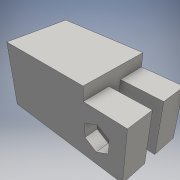
# Autodesk Inventor part: connectiontest1
Saved by Autodesk Inventor 2016 (Build 200138000, 138)
## iProperties
Created: 2015-11-19
Part Number: connectiontest1
Material: Generic
Document SubType Name: Modeling
Designer: hesaon
Density: 1 g/cm^3
Appearance: Default
Author: hesaon
Autodesk Inventor part; units mm, degrees
ref_plane "YZ Plane" through (0, 0, 0) normal (1, 0, 0) x (0, 1, 0)
ref_plane "XZ Plane" through (0, 0, 0) normal (0, 1, 0) x (-1, 0, 0)
ref_plane "XY Plane" through (0, 0, 0) normal (0, 0, 1) x (1, 0, 0)
sketch "Sketch1" plane through (0, 0, 0) normal (0, 0, 1) x (1, 0, 0)
  line L0 (0, 0) -> (-40, 0)
  line L1 (-40, 0) -> (-40, 20)
  line L2 (-40, 20) -> (0, 20)
  line L3 (0, 20) -> (0, 0)
  dimension "d0" = 40
  dimension "d1" = 20
  constraints: 8 end point, 2 parallel, 1 horizontal, 1 perpendicular
  measures "d0" distance of L1.end L2.end
  measures "d1" distance of L0.end L1.end
extrude "Extrusion1" add sketch "Sketch1" along normal blind 20
sketch "Sketch2" plane through (-40, 20, 0) normal (0, 1, 0) x (1, 0, 0)
  line L0 (0, -20) -> (40, -20) projected
  line L1 (40, -20) -> (40, -16)
  line L2 (40, 0) -> (40, -20) projected
  line L3 (28, -20) -> (28, -16)
  line L4 (28, -16) -> (40, -16)
  dimension "d4" = 4
  dimension "d5" = 12
  constraints: 6 end point, 2 point on line, 1 perpendicular, 1 vertical
  measures "d4" distance of L0.end L1.end
  measures "d5" distance of L1.end L3.end
extrude "Extrusion2" cut sketch "Sketch2" against normal through all
sketch "Sketch3" plane through (0, 0, 0) normal (1, 0, 0) x (0, 0, -1)
  line L0 (-16, 20) -> (-16, 0) projected
  line L1 (-16, 12) -> (0, 12)
  line L2 (0, 20) -> (0, 0) projected
  line L3 (0, 8) -> (-16, 8)
  dimension "d8" = 8
  dimension "d9" = 8
  constraints: 4 end point, 4 point on line, 1 horizontal, 1 parallel
  measures "d8" distance of L2.start L1.end
  measures "d9" distance of L2.end L3.start
extrude "Extrusion3" cut sketch "Sketch3" against normal blind 12
sketch "Sketch4" plane through (-40, 20, 0) normal (0, 1, 0) x (1, 0, 0)
  circle A0 centre (32, -8) radius 2.25
  line L0 (28, -16) -> (40, -16) projected
  line L1 (40, 0) -> (40, -16) projected
  dimension "d12" = 4.5
  dimension "d13" = 8
  dimension "d14" = 8
  constraints: 1 centre point
  measures "d12" diameter of A0
  measures "d13" distance from line of L0 A0.centre
  measures "d14" distance from line of A0.centre L1
extrude "Extrusion4" cut sketch "Sketch4" against normal through all
sketch "Sketch5" plane through (-40, 0, 0) normal (0, -1, 0) x (1, 0, 0)
  line L0 (40, 0) -> (40, 16) projected
  line L1 (0, 0) -> (0, 20) projected
  line L2 (40, 0) -> (32, 0)
  line L3 (32, 12.1569) -> (35.6, 10.0785)
  line L4 (35.6, 10.0785) -> (35.6, 5.9215)
  line L5 (35.6, 5.9215) -> (32, 3.8431)
  line L6 (32, 3.8431) -> (28.4, 5.9215)
  line L7 (28.4, 5.9215) -> (28.4, 10.0785)
  line L8 (28.4, 10.0785) -> (32, 12.1569)
  line L9 (40, 16) -> (28, 16) projected
  dimension "d28" = 7.2
  dimension "d29" = 4.4
  dimension "d30" = 3.8431
  dimension "d31" = 3.8431
  dimension "d32" = 2.0785
  dimension "d33" = 4.1569
  dimension "d34" = 2.0785
  constraints: 14 end point
  measures "d28" distance between parallel lines of L4 L7
  measures "d29" distance between parallel lines of L0 L4
  measures "d30" distance of L2.end L5.end
  measures "d31" distance from line of L9 L3.start
  measures "d32" vertical distance of L3.end L3.start
  measures "d33" distance of L3.end L4.end
  measures "d34" vertical distance of L4.end L5.end
extrude "Extrusion5" cut sketch "Sketch5" against normal blind 4
sketch "Sketch6" plane through (-40, 20, 0) normal (0, 1, 0) x (1, 0, 0)
  circle A0 centre (32, -8) radius 4
  line L0 (28, -16) -> (40, -16) projected
  line L1 (40, 0) -> (40, -16) projected
  dimension "d37" = 8
  dimension "d38" = 8
  dimension "d39" = 8
  constraints: 1 centre point
  measures "d37" diameter of A0
  measures "d38" distance from line of L0 A0.centre
  measures "d39" distance from line of L1 A0.centre
extrude "Extrusion6" cut sketch "Sketch6" against normal blind 4
body "Solid1"
